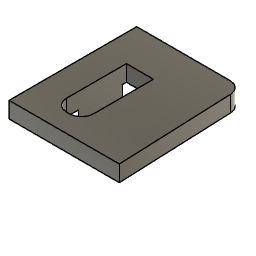
SNES - Front Cutting Tool v12 (Autodesk Fusion 360 design; units mm, degrees)
Autodesk Fusion 360 part; units mm, degrees
sketch "Boceto1" plane through (0, 0, 0) normal (0, 0, 1) x (1, 0, 0)
  circle A0 centre (0, 0) radius 3.2
  line L0 (-5, 7.8) -> (8, 7.8)
  line L1 (8.65, -8) -> (-5, -8)
  line L2 (-5, -8) -> (-5, 7.8)
  line L3 (8, 7.8) -> (8.65, -8)
  line L4 (-1.675, 3.2) -> (1.675, 3.2)
  line L5 (1.675, 3.2) -> (1.675, -5.7)
  line L6 (1.675, -5.7) -> (-1.675, -5.7)
  line L7 (-1.675, -5.7) -> (-1.675, 3.2)
  dimension "d1" = 6.4
  dimension "d6" = 7.8
  dimension "d7" = 8
  dimension "d14" = 8
  dimension "d16" = 3.35
  dimension "d17" = 1.675
  dimension "d18" = 5.7
  dimension "d24" = 8.65
  dimension "d27" = 3.2
  dimension "d28" = 5
  constraint coincident A0.centre origin
  constraint horizontal L0
  constraint horizontal L1
  constraint vertical L2
  constraint horizontal L4
  constraint vertical L5
  constraint horizontal L6
  constraint vertical L7
  measures "d1" diameter of A0
  measures "d6" vertical distance of A0.centre L0.end
  measures "d7" vertical distance of A0.centre L1.end
  measures "d14" horizontal distance of A0.centre L0.end
  measures "d16" distance of L4.start L4.end
  measures "d17" horizontal distance of A0.centre L4.start
  measures "d18" vertical distance of A0.centre L6.end
  measures "d24" horizontal distance of A0.centre L1.start
  measures "d27" vertical distance of A0.centre L4.start
  measures "d28" horizontal distance of A0.centre L0.start
extrude "Extruir1" add sketch "Boceto1" against normal blind 1 contours A0 L4 L5 | A0 L5 L6 L7 | A0 L4 L7 | L0 L1 L2 L3
extrude "Extruir2" add sketch "Boceto1" against normal blind 6 contours A0 L5 | A0 L5 L7 | A0 L7
fillet "Empalme1" radius 0.5 1 edges at (-2.9834, 1.1572, -6)
extrude "Extruir3" cut sketch "Boceto1" against normal blind 10 contours A0 L5 L7 | A0 L4 L5 | A0 L5 L6 L7 | A0 L4 L7
fillet "Empalme2" radius 1.5 2 edges at (1.675, -5.7, -0.5) (-1.675, -5.7, -0.5)
fillet "Empalme3" radius 1.5 1 edges at (8, 7.8, -0.5)
extrude "Extruir4" add 1 faces at (6.1281, -1.9461, 0) along direction (0, 0, 1) blind 1
equation "d2 = d1 + ( ( 2 * 1 ) * 1 mm )"
equation "d6 = ( d1 / 2 ) + 4.6 mm"
equation "d14 = ( d1 / 2 ) + 4.8 mm"
equation "d17 = d16 / 2"
equation "d18 = d1 / 2 + 2.5 mm"
equation "d27 = d1 / 2"
